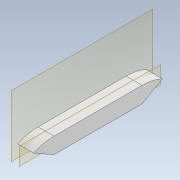
# Autodesk Inventor part: Tractive Light Enclosure 2.0
Saved by Autodesk Inventor 2021 (Build 250183000, 183)
## iProperties
Created: 2020-10-01
Part Number: Tractive Light Enclosure 2.0
Material: Generic
Document SubType Name: Modeling
Designer: capta
Density: 1 g/cm^3
Appearance: Default
Author: capta
Autodesk Inventor part; units mm, degrees
ref_plane "XZ Plane" through (0, 0, 0) normal (0, 1, 0) x (-1, 0, 0)
sketch "Sketch1" plane through (0, 0, 0) normal (1, 0, 0) x (0, 1, 0)
  line L0 (0, 0) -> (0, -139.7)
  arc A0 (-25.4, 0) -> (-101.6, 76.2) centre (-101.6, 0) ccw
  line L1 (-101.6, 0) -> (-25.4, 0)
  line L2 (-25.4, 0) -> (-25.4, -139.7)
  arc A1 (0, 0) -> (-101.6, 101.6) centre (-101.6, 0) ccw
  line L3 (-101.6, 76.2) -> (-101.6, 101.6)
  line L4 (0, -69.85) -> (10.3155, -69.85)
  arc A2 (-101.6, -215.9) -> (-25.4, -139.7) centre (-101.6, -139.7) ccw
  arc A3 (-101.6, -241.3) -> (0, -139.7) centre (-101.6, -139.7) ccw
  line L5 (-101.6, -215.9) -> (-101.6, -241.3)
  line L6 (-25.4, -69.85) -> (-50.8, -69.85)
  line L7 (-50.8, -69.85) -> (-50.8, 0)
  line L8 (-50.8, 0) -> (-32.5333, 32.1905)
  line L9 (-50.8, -69.85) -> (-50.8, -139.7)
  line L10 (-50.8, -139.7) -> (-32.5333, -171.8905)
  dimension "d0" = 139.7
  dimension "d2" = 152.4
  dimension "d3" = 25.4
  dimension "d4" = 25.4
  constraints: 22 end point, 10 point on circle, 4 centre point, 2 coincident, 2 midpoint, 2 point on line, 2 symmetric about line, 1 horizontal, 1 perpendicular
  measures "d0" distance of L0.start L0.end
  measures "d2" diameter of A0
  measures "d3" distance between parallel lines of L0 L2
  measures "d4" distance of L6.start L6.end
extrude "Extrusion1" add sketch "Sketch1" along normal blind 25.4 contours A0 L1 L8 | L2 L6 L7 L1 | L10 L9 L6 L2 A2
ref_plane "Work Plane1" through (12.7, 0, 0) normal (1, 0, 0) x (0, 0, -1)
body "Solid1"
